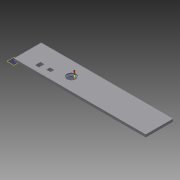
# Autodesk Inventor part: placa laterala usb
Saved by Autodesk Inventor 2015 SP1 (Build 190203100, 203)
## iProperties
Created: 2015-05-04
Part Number: placa laterala usb
Material: Generic
Document SubType Name: Modeling
Designer: ubik
Density: 1 g/cm^3
Appearance: Default
Author: ubik
Autodesk Inventor part; units mm, degrees
ref_plane "YZ Plane" through (0, 0, 0) normal (1, 0, 0) x (0, 1, 0)
ref_plane "XZ Plane" through (0, 0, 0) normal (0, 1, 0) x (-1, 0, 0)
ref_plane "XY Plane" through (0, 0, 0) normal (0, 0, 1) x (1, 0, 0)
sketch "Sketch1" plane through (0, 0, 0) normal (0, 0, 1) x (1, 0, 0)
  line L0 (0, 0) -> (415, 0)
  line L1 (415, 0) -> (415, 86)
  line L2 (415, 86) -> (0, 86)
  line L3 (0, 86) -> (0, 0)
  line L4 (82, 32) -> (95, 32)
  line L5 (95, 32) -> (95, 20.5)
  line L6 (95, 20.5) -> (82, 20.5)
  line L7 (82, 20.5) -> (82, 32)
  line L8 (52, 32) -> (64, 32)
  line L9 (64, 32) -> (64, 15)
  line L10 (64, 15) -> (52, 15)
  line L11 (52, 15) -> (52, 32)
  circle A0 centre (140, 41) radius 11
  dimension "d0" = 415
  dimension "d1" = 86
  dimension "d2" = 82
  dimension "d3" = 54
  dimension "d4" = 13
  dimension "d5" = 11.5
  dimension "d8" = 18
  dimension "d9" = 12
  dimension "d10" = 17
  dimension "d11" = 54
  dimension "d12" = 22
  dimension "d13" = 45
  dimension "d14" = 45
  constraints: 24 end point, 6 parallel, 3 horizontal, 3 perpendicular, 1 centre point
  measures "d0" distance of L2.end L1.end
  measures "d1" distance of L1.end L0.end
  measures "d2" distance between parallel lines of L3 L7
  measures "d3" distance between parallel lines of L2 L4
  measures "d4" distance of L4.start L4.end
  measures "d5" distance of L4.end L5.end
  measures "d8" distance between parallel lines of L7 L9
  measures "d9" distance of L8.start L8.end
  measures "d10" distance of L10.end L8.start
  measures "d11" distance between parallel lines of L2 L8
  measures "d12" diameter of A0
  measures "d13" distance from line of A0.centre L5
  measures "d14" distance from line of A0.centre L2
ref_plane "Work Plane1" through (0, 0, 0) normal (0, 0, -1) x (-1, 0, 0)
extrude "Extrusion2" add sketch "Sketch1" along normal blind 8
hole "Hole1" at (140, 41, 8) direction (0, 0, -1) diameter 29 depth 4 tip angle 118
body "Solid2"
